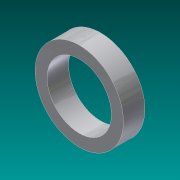
# Autodesk Inventor part: 膝_同軸_スペーサ_1_1
Saved by Autodesk Inventor 2015 (Build 190159000, 159)
## iProperties
Created: 2016-05-01
Part Number: 膝_同軸_スペーサ_1_1
Material: アルミニウム 2014-T4
Document SubType Name: Modeling
Designer: hiroaki
Density: 2.8 g/cm^3
Appearance: サテン
Mass: 0.0910038 g
Surface Area: 1.04536 cm^2
Volume: 0.0325013 cm^3
Author: hiroaki
Autodesk Inventor part; units mm, degrees
ref_plane "YZ Plane" through (0, 0, 0) normal (1, 0, 0) x (0, 1, 0)
ref_plane "XZ Plane" through (0, 0, 0) normal (0, 1, 0) x (-1, 0, 0)
ref_plane "XY Plane" through (0, 0, 0) normal (0, 0, 1) x (1, 0, 0)
sketch "スケッチ1" plane through (0, 0, 0) normal (0, 0, 1) x (1, 0, 0)
  line L0 (2.55, 0.85) -> (2.55, -0.85)
  line L1 (2.55, -0.85) -> (3.5, -0.85)
  line L2 (3.5, -0.85) -> (3.5, 0.85)
  line L3 (3.5, 0.85) -> (2.55, 0.85)
  line L4 (0, -1.19) -> (0, 1.19) projected
  point P0 (0, 0)
  point P1 (2.55, 0)
  dimension "d0" = 2.55
  dimension "d3" = 3.5
  dimension "d4" = 1.7
  constraints: 8 end point, 3 perpendicular, 1 horizontal alignment, 1 midpoint, 1 vertical
  measures "d0" distance from line of L0 point (0, 0)
  measures "d3" distance from line of L2 point (0, 0)
  measures "d4" distance of L1.end L2.end
revolve "回転1" add sketch "スケッチ1" angle 360 about axis through (0, -10, 0) along (0, 1, 0)
